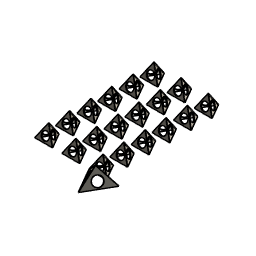
day15-painters-tripod (Autodesk Fusion 360 design; units mm, degrees)
part number: 2025-06-27-20-24-31-571
part number: 2025-06-27-20-27-47-141
part number: 2025-06-27-20-44-16-772
Autodesk Fusion 360 part; units mm, degrees
sketch "Sketch1" plane through (0, 0, 0) normal (0, 0, 1) x (1, 0, 0) in component "60mm painter's tripod"
  line L0 (0, 0) -> (30, 51.9615)
  line L1 (30, 51.9615) -> (60, 0)
  line L2 (60, 0) -> (0, 0)
  dimension "d1" = 60
  constraint coincident L0.start L2.end
  constraint horizontal L2
  constraint equal L0 L1
  constraint equal L1 L2
  measures "d1" distance of L0.start L0.end
ref_plane "WorkPlane1" through (0, 0, 50) normal (0, 0, 1) x (1, 0, 0) in component "60mm painter's tripod"
sketch "Sketch2" plane through (0, 0, 50) normal (0, 0, 1) x (1, 0, 0) in component "60mm painter's tripod"
  line L0 (0, 0) -> (30, 51.9615)
  line L1 (30, 51.9615) -> (60, 0)
  line L2 (60, 0) -> (0, 0)
  line L3 (30, 51.9615) -> (30, 0) construction
  line L4 (0, 0) -> (45, 25.9808) construction
  point P0 (30, 17.3205)
  constraint coincident L0.end L1.start
  constraint midpoint L2 L3.end
  constraint coincident L0.start L2.end
  constraint midpoint L1 L4.end
  constraint coincident L3 P0
  constraint coincident L4 P0
loft "Loft1" add profiles "Sketch1" section 1 section 2 point at (30, 17.3205, 50) makes body 1 in component "60mm painter's tripod"
shell "Shell1" thickness 2.5 removed faces 1 at (30, 17.3205, 0) on bodies 1 in component "60mm painter's tripod"
sketch "Sketch3" plane through (0, 0, 0) normal (0, -0.944911, 0.327327) x (1, 0, 0) in component "60mm painter's tripod"
  line L0 (0, 0) -> (60, 0)
  line L1 (60, 0) -> (30, 52.915)
  line L2 (30, 52.915) -> (0, 0)
  line L3 (30, 52.915) -> (30, 0) construction
  line L4 (0, 0) -> (45, 26.4575) construction
  circle A0 centre (30, 17.6383) radius 12.5
  dimension "d4" = 25
  constraint coincident L1.end L2.start
  constraint perpendicular L0 L3
  constraint midpoint L0 L3.end
  constraint coincident L0.start L2.end
  constraint midpoint L1 L4.end
  constraint coincident L3 A0.centre
  constraint coincident L4 A0.centre
  measures "d4" diameter of A0
extrude "Extrude1" cut sketch "Sketch3" against normal blind 2.5 contours A0 bodies 1 in component "60mm painter's tripod"
pattern_circular "C-Pattern1" count 3 over 360 about axis through (30, 17.3205, 75) along (0, 0, -1) of "Extrude1" in component "60mm painter's tripod"
fillet "Fillet1" radius 0.5 6 edges at (45, 8.6603, 25) (30, 34.641, 25) (15, 8.6603, 25) (18.3459, 7.2531, 20.9378) (44.5457, 12.2615, 20.9378) (27.1084, 32.447, 20.9378) on bodies 1 in component "60mm painter's tripod"
sketch "Sketch1 (2)" plane through (0, 0, 0) normal (0, 0, 1) x (1, 0, 0) in component "60mm painter's tripod (1)"
  line L0 (0, 0) -> (50, 86.6025)
  line L1 (50, 86.6025) -> (100, 0)
  line L2 (100, 0) -> (0, 0)
  dimension "d1_1" = 100
  constraint coincident L0.start L2.end
  constraint horizontal L2
  constraint equal L0 L1
  constraint equal L1 L2
  measures "d1_1" distance of L0.start L0.end
ref_plane "WorkPlane1" through (0, 0, 50) normal (0, 0, 1) x (1, 0, 0) in component "60mm painter's tripod (1)"
sketch "Sketch2 (2)" plane through (0, 0, 50) normal (0, 0, 1) x (1, 0, 0) in component "60mm painter's tripod (1)"
  line L0 (0, 0) -> (50, 86.6025)
  line L1 (50, 86.6025) -> (100, 0)
  line L2 (100, 0) -> (0, 0)
  line L3 (50, 86.6025) -> (50, 0) construction
  line L4 (0, 0) -> (75, 43.3013) construction
  point P0 (50, 28.8675)
  constraint coincident L0.end L1.start
  constraint midpoint L2 L3.end
  constraint coincident L0.start L2.end
  constraint midpoint L1 L4.end
  constraint coincident L3 P0
  constraint coincident L4 P0
loft "Loft1'" add profiles "Sketch1 (2)" section 1 section 2 point at (50, 28.8675, 50) separate body makes body 2 in component "60mm painter's tripod (1)"
shell "Shell1'" thickness 2.5 removed faces 1 at (50, 28.8675, 0) on bodies 2 in component "60mm painter's tripod (1)"
sketch "Sketch3 (2)" plane through (0, 0, 0) normal (0, -0.866025, 0.5) x (1, 0, 0) in component "60mm painter's tripod (1)"
  line L0 (0, 0) -> (100, 0)
  line L1 (100, 0) -> (50, 57.735)
  line L2 (50, 57.735) -> (0, 0)
  line L3 (50, 57.735) -> (50, 0) construction
  line L4 (0, 0) -> (75, 28.8675) construction
  circle A0 centre (50, 19.245) radius 15
  dimension "d4_1" = 30
  constraint coincident L1.end L2.start
  constraint perpendicular L0 L3
  constraint midpoint L0 L3.end
  constraint coincident L0.start L2.end
  constraint midpoint L1 L4.end
  constraint coincident L3 A0.centre
  constraint coincident L4 A0.centre
  measures "d4_1" diameter of A0
extrude "Extrude1'" cut sketch "Sketch3 (2)" against normal blind 2.5 contours A0 bodies 2 in component "60mm painter's tripod (1)"
pattern_circular "C-Pattern1'" count 3 over 360 about axis through (50, 28.8675, 125) along (0, 0, -1) of "Extrude1'" in component "60mm painter's tripod (1)"
fillet "Fillet1'" radius 0.5 6 edges at (75, 14.4338, 25) (50, 57.735, 25) (25, 14.4338, 25) (36.0151, 12.3346, 21.3642) (71.3104, 25.0227, 21.3642) (42.6745, 49.2452, 21.3642) on bodies 2 in component "60mm painter's tripod (1)"
pattern_linear "00000000-0000-0000-0000-000000000000" [suppressed]
component "60mm painter's tripod" placed x (1, 0, 0) y (0, 1, 0) z (0, 0, 1) at (0, 0, 0)
component "60mm painter's tripod" placed x (1, 0, 0) y (0, 1, 0) z (0, 0, 1) at (0, 69, 0)
component "60mm painter's tripod (1)" placed x (0.5, -0.866025, 0) y (0.866025, 0.5, 0) z (0, 0, 1) at (0.4433, 0.6495, 0)
component "60mm painter's tripod" placed x (1, 0, 0) y (0, 1, 0) z (0, 0, 1) at (0, 209, 0)
component "60mm painter's tripod" placed x (1, 0, 0) y (0, 1, 0) z (0, 0, 1) at (0, 140, 0)
component "60mm painter's tripod" placed x (1, 0, 0) y (0, 1, 0) z (0, 0, 1) at (0, 349, 0)
component "60mm painter's tripod" placed x (1, 0, 0) y (0, 1, 0) z (0, 0, 1) at (0, 280, 0)
component "60mm painter's tripod" placed x (1, 0, 0) y (0, 1, 0) z (0, 0, 1) at (-90, 69, 0)
component "60mm painter's tripod" placed x (1, 0, 0) y (0, 1, 0) z (0, 0, 1) at (-90, 0, 0)
component "60mm painter's tripod" placed x (1, 0, 0) y (0, 1, 0) z (0, 0, 1) at (-90, 209, 0)
component "60mm painter's tripod" placed x (1, 0, 0) y (0, 1, 0) z (0, 0, 1) at (-90, 140, 0)
component "60mm painter's tripod" placed x (1, 0, 0) y (0, 1, 0) z (0, 0, 1) at (-90, 349, 0)
component "60mm painter's tripod" placed x (1, 0, 0) y (0, 1, 0) z (0, 0, 1) at (-90, 280, 0)
component "60mm painter's tripod" placed x (1, 0, 0) y (0, 1, 0) z (0, 0, 1) at (-180, 69, 0)
component "60mm painter's tripod" placed x (1, 0, 0) y (0, 1, 0) z (0, 0, 1) at (-180, 0, 0)
component "60mm painter's tripod" placed x (1, 0, 0) y (0, 1, 0) z (0, 0, 1) at (-180, 209, 0)
component "60mm painter's tripod" placed x (1, 0, 0) y (0, 1, 0) z (0, 0, 1) at (-180, 140, 0)
component "60mm painter's tripod" placed x (1, 0, 0) y (0, 1, 0) z (0, 0, 1) at (-180, 349, 0)
component "60mm painter's tripod" placed x (1, 0, 0) y (0, 1, 0) z (0, 0, 1) at (-180, 280, 0)
